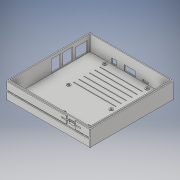
# Autodesk Inventor part: Tray
Saved by Autodesk Inventor 2018 (Build 220112000, 112)
## iProperties
Created: 2019-05-02
Part Number: Tray
Material: Generic
Document SubType Name: Modeling
Designer: thatg
Density: 1 g/cm^3
Appearance: Default
Author: thatg
Autodesk Inventor part; units mm, degrees
ref_plane "YZ Plane" through (0, 0, 0) normal (1, 0, 0) x (0, 1, 0)
ref_plane "XZ Plane" through (0, 0, 0) normal (0, 1, 0) x (-1, 0, 0)
ref_plane "XY Plane" through (0, 0, 0) normal (0, 0, 1) x (1, 0, 0)
sketch "Sketch1" plane through (0, 0, 0) normal (0, 1, 0) x (-1, 0, 0)
  line L0 (-57.15, 57.15) -> (57.15, 57.15)
  line L1 (57.15, 57.15) -> (57.15, -57.15)
  line L2 (57.15, -57.15) -> (-57.15, -57.15)
  line L3 (-57.15, -57.15) -> (-57.15, 57.15)
  line L4 (-57.15, 57.15) -> (57.15, -57.15) construction
  line L5 (57.15, 57.15) -> (-57.15, -57.15) construction
  point P0 (0, 0)
  dimension "d0" = 114.3
  dimension "d1" = 114.3
  constraints: 12 end point, 2 midpoint, 2 parallel, 1 horizontal, 1 perpendicular
  measures "d0" distance of L1.end L2.end
  measures "d1" distance of L0.end L1.end
extrude "Extrusion1" add sketch "Sketch1" along normal blind 2.54
sketch "Sketch4" plane through (0, 2.54, 0) normal (0, 1, 0) x (1, 0, 0)
  line L0 (-57.15, -57.15) -> (57.15, -57.15) projected
  line L1 (57.15, -57.15) -> (57.15, 57.15) projected
  line L2 (57.15, 57.15) -> (-57.15, 57.15) projected
  line L3 (-57.15, 57.15) -> (-57.15, -57.15) projected
  line L4 (-54.61, 54.61) -> (54.61, 54.61)
  line L5 (54.61, 54.61) -> (54.61, -54.61)
  line L6 (54.61, -54.61) -> (-54.61, -54.61)
  line L7 (-54.61, -54.61) -> (-54.61, 54.61)
  point P0 (0, 0)
  dimension "d11" = 2.54
  constraints: 8 end point, 3 other
  measures "d11" distance between parallel lines of L2 L4
extrude "Extrusion4" add sketch "Sketch4" along normal blind 20
sketch "Sketch6" plane through (0, 2.54, 0) normal (0, 1, 0) x (1, 0, 0)
  line L0 (-53.34, 53.34) -> (-53.34, -0.12)
  line L1 (-53.34, 53.34) -> (-53.34, -2.66)
  line L2 (-53.34, -2.66) -> (31.66, -2.66)
  line L3 (31.66, -2.66) -> (31.66, 53.34)
  line L4 (31.66, 53.34) -> (-53.34, 53.34)
  line L5 (-53.34, 53.34) -> (31.66, 53.34)
  line L6 (31.66, 53.34) -> (31.66, -2.66)
  line L7 (31.66, -2.66) -> (-53.34, -2.66)
  line L8 (-53.34, -2.66) -> (-53.34, 53.34)
  line L9 (-57.15, 8.34) -> (-54.61, 8.34)
  line L10 (-57.15, 24.34) -> (-54.61, 24.34)
  line L11 (-57.15, 43.09) -> (-54.61, 43.09)
  line L12 (-57.15, 53.34) -> (-53.34, 53.34)
  line L13 (-57.15, 14.915) -> (-54.61, 14.915)
  line L14 (-57.15, 1.765) -> (-54.61, 1.765)
  line L15 (-57.15, 30.915) -> (-54.61, 30.915)
  line L16 (-57.15, 17.765) -> (-54.61, 17.765)
  line L17 (-57.15, 51.065) -> (-54.61, 51.065)
  line L18 (-57.15, 35.115) -> (-54.61, 35.115)
  line L19 (-57.15, 51.065) -> (-54.61, 51.065)
  line L20 (-53.34, 51.065) -> (-53.34, 35.115)
  line L21 (-54.61, 35.115) -> (-57.15, 35.115)
  line L22 (-57.15, 35.115) -> (-57.15, 51.065)
  line L23 (-57.15, 30.915) -> (-54.61, 30.915)
  line L24 (-53.34, 30.915) -> (-53.34, 17.765)
  line L25 (-54.61, 17.765) -> (-57.15, 17.765)
  line L26 (-57.15, 17.765) -> (-57.15, 30.915)
  line L27 (-57.15, 14.915) -> (-54.61, 14.915)
  line L28 (-53.34, 14.915) -> (-53.34, 1.765)
  line L29 (-54.61, 1.765) -> (-57.15, 1.765)
  line L30 (-57.15, 1.765) -> (-57.15, 14.915)
  line L31 (31.66, 53.34) -> (31.66, 57.15)
  line L32 (21.06, 57.15) -> (21.06, 54.61)
  line L33 (17.06, 57.15) -> (17.06, 54.61)
  line L34 (25.06, 57.15) -> (25.06, 54.61)
  line L35 (-0.34, 57.15) -> (-0.34, 54.61)
  line L36 (7.41, 57.15) -> (7.41, 54.61)
  line L37 (-8.09, 57.15) -> (-8.09, 54.61)
  line L38 (-21.84, 57.15) -> (-21.84, 54.61)
  line L39 (-25.09, 57.15) -> (-25.09, 54.61)
  line L40 (-18.59, 57.15) -> (-18.59, 54.61)
  line L41 (-25.09, 57.15) -> (-18.59, 57.15)
  line L42 (-18.59, 57.15) -> (-18.59, 54.61)
  line L43 (-18.59, 53.34) -> (-25.09, 53.34)
  line L44 (-25.09, 54.61) -> (-25.09, 57.15)
  line L45 (-8.09, 57.15) -> (7.41, 57.15)
  line L46 (7.41, 57.15) -> (7.41, 54.61)
  line L47 (7.41, 53.34) -> (-8.09, 53.34)
  line L48 (-8.09, 54.61) -> (-8.09, 57.15)
  line L49 (17.06, 57.15) -> (25.06, 57.15)
  line L50 (25.06, 57.15) -> (25.06, 54.61)
  line L51 (25.06, 53.34) -> (17.06, 53.34)
  line L52 (17.06, 54.61) -> (17.06, 57.15)
  line L53 (-54.61, 54.61) -> (54.61, 54.61) projected
  line L54 (-25.09, 54.61) -> (-18.59, 54.61)
  line L55 (-8.09, 54.61) -> (7.41, 54.61)
  line L56 (17.06, 54.61) -> (25.06, 54.61)
  line L57 (-54.61, -54.61) -> (-54.61, 54.61) projected
  line L58 (-54.61, 51.065) -> (-54.61, 35.115)
  line L59 (-54.61, 30.915) -> (-54.61, 17.765)
  line L60 (-54.61, 14.915) -> (-54.61, 1.765)
  point P0 (0, 0)
  dimension "d17" = 56
  dimension "d18" = 85
  dimension "d21" = 10.25
  dimension "d22" = 18.75
  dimension "d23" = 16
  dimension "d24" = 6.575
  dimension "d25" = 6.575
  dimension "d26" = 6.575
  dimension "d27" = 6.575
  dimension "d28" = 7.975
  dimension "d29" = 7.975
  dimension "d30" = 10.6
  dimension "d31" = 4
  dimension "d32" = 4
  dimension "d33" = 21.4
  dimension "d34" = 7.75
  dimension "d35" = 7.75
  dimension "d37" = 21.5
  dimension "d38" = 3.25
  dimension "d39" = 3.25
  constraints: 118 end point, 26 parallel, 15 perpendicular, 9 horizontal, 6 point on line, 5 midpoint, 1 vertical, 8 other
  measures "d17" distance of L0.start L1.end
  measures "d18" distance of L1.end L2.end
  measures "d21" distance of L12.start L11.start
  measures "d22" distance of L11.start L10.start
  measures "d23" distance of L10.start L9.start
  measures "d24" distance between parallel lines of L9 L13
  measures "d25" distance between parallel lines of L9 L14
  measures "d26" distance between parallel lines of L10 L15
  measures "d27" distance between parallel lines of L10 L16
  measures "d28" distance between parallel lines of L11 L17
  measures "d29" distance between parallel lines of L11 L18
  measures "d30" distance of L31.end L32.start
  measures "d31" distance between parallel lines of L32 L33
  measures "d32" distance between parallel lines of L32 L34
  measures "d33" distance of L32.start L35.start
  measures "d34" distance between parallel lines of L35 L36
  measures "d35" distance between parallel lines of L35 L37
  measures "d37" distance of L35.start L38.start
  measures "d38" distance between parallel lines of L38 L39
  measures "d39" distance between parallel lines of L38 L40
extrude "Extrusion5" cut sketch "Sketch6" along normal blind 17.5 contours L30 L13 L57 L9 | L9 L57 L14 L30 | L26 L15 L57 L10 | L10 L57 L16 L26
extrude "Extrusion6" cut sketch "Sketch6" along normal blind 15 contours L22 L17 L57 L11 | L11 L57 L18 L22
extrude "Extrusion7" cut sketch "Sketch6" along normal blind 7.5 contours L39 L41 L38 L53 | L38 L41 L40 L53
extrude "Extrusion8" cut sketch "Sketch6" along normal blind 8 contours L37 L45 L35 L53 | L35 L45 L36 L53
extrude "Extrusion9" cut sketch "Sketch6" along normal blind 3.5 contours L53 L32 L49 L34 | L33 L49 L32 L53
sketch "Sketch7" plane through (0, 2.54, 0) normal (0, 1, 0) x (1, 0, 0)
  line L0 (-57.15, 1.765) -> (-57.15, 14.915) projected
  line L1 (-57.15, 1.765) -> (-54.61, 1.765) projected
  line L2 (-54.61, 14.915) -> (-57.15, 14.915) projected
  line L3 (-57.15, 17.765) -> (-54.61, 17.765) projected
  line L4 (-57.15, 17.765) -> (-57.15, 30.915) projected
  line L5 (-54.61, 30.915) -> (-57.15, 30.915) projected
  line L6 (-57.15, 35.115) -> (-54.61, 35.115) projected
  line L7 (-57.15, 35.115) -> (-57.15, 51.065) projected
  line L8 (-54.61, 51.065) -> (-57.15, 51.065) projected
  line L9 (-18.59, 54.61) -> (-18.59, 57.15) projected
  line L10 (-25.09, 57.15) -> (-18.59, 57.15) projected
  line L11 (-25.09, 57.15) -> (-25.09, 54.61) projected
  line L12 (-8.09, 57.15) -> (-8.09, 54.61) projected
  line L13 (-8.09, 57.15) -> (7.41, 57.15) projected
  line L14 (7.41, 54.61) -> (7.41, 57.15) projected
  line L15 (17.06, 57.15) -> (17.06, 54.61) projected
  line L16 (17.06, 57.15) -> (25.06, 57.15) projected
  line L17 (25.06, 54.61) -> (25.06, 57.15) projected
  line L18 (-54.61, 1.765) -> (-54.61, 14.915)
  line L19 (-54.61, 17.765) -> (-54.61, 30.915)
  line L20 (-54.61, 35.115) -> (-54.61, 51.065)
  line L21 (-25.09, 54.61) -> (-18.59, 54.61)
  line L22 (-8.09, 54.61) -> (7.41, 54.61)
  line L23 (17.06, 54.61) -> (25.06, 54.61)
  point P0 (0, 0)
  constraints: 12 end point, 4 collinear, 1 perpendicular, 1 vertical
extrude "Extrusion10" add sketch "Sketch7" along normal blind 1
sketch "Sketch8" plane through (0, 2.54, 0) normal (0, 1, 0) x (1, 0, 0)
  line L0 (-53.34, -2.66) -> (31.66, -2.66) projected
  line L1 (31.66, -2.66) -> (31.66, 53.34) projected
  line L2 (31.66, 53.34) -> (-53.34, 53.34) projected
  line L3 (-53.34, 53.34) -> (-53.34, -2.66) projected
  line L4 (31.66, -2.66) -> (28.16, -2.66)
  line L5 (28.16, -2.66) -> (28.16, 0.84)
  circle A0 centre (28.16, 0.84) radius 1.175
  line L6 (31.66, 53.34) -> (28.16, 53.34)
  line L7 (28.16, 53.34) -> (28.16, 49.84)
  circle A1 centre (28.16, 49.84) radius 1.175
  line L8 (28.16, 0.84) -> (-29.84, 0.84)
  circle A2 centre (-29.84, 0.84) radius 1.175
  line L9 (28.16, 49.84) -> (-29.84, 49.84)
  circle A3 centre (-29.84, 49.84) radius 1.175
  circle A4 centre (-29.84, 0.84) radius 2.445
  circle A5 centre (28.16, 0.84) radius 2.445
  circle A6 centre (28.16, 49.84) radius 2.445
  circle A7 centre (-29.84, 49.84) radius 2.445
  point P0 (0, 0)
  dimension "d52" = 3.5
  dimension "d53" = 3.5
  dimension "d54" = 2.35
  dimension "d56" = 3.5
  dimension "d57" = 3.5
  dimension "d58" = 2.35
  dimension "d59" = 58
  dimension "d60" = 2.35
  dimension "d61" = 58
  dimension "d62" = 2.35
  dimension "d63" = 1.27
  dimension "d64" = 1.27
  dimension "d65" = 1.27
  dimension "d66" = 1.27
  constraints: 12 end point, 8 centre point, 4 coincident, 2 perpendicular, 2 point on line, 1 horizontal, 1 parallel
  measures "d52" distance of L0.end L4.end
  measures "d53" distance of L4.end L5.end
  measures "d54" diameter of A0
  measures "d56" distance of L1.end L6.end
  measures "d57" distance of L6.end L7.end
  measures "d58" diameter of A1
  measures "d59" distance of L8.start L8.end
  measures "d60" diameter of A2
  measures "d61" distance of L9.start L9.end
  measures "d62" diameter of A3
  measures "d63" radial gap between concentric circles of A2 A4
  measures "d64" radial gap between concentric circles of A0 A5
  measures "d65" radial gap between concentric circles of A1 A6
  measures "d66" radial gap between concentric circles of A3 A7
extrude "Extrusion11" add sketch "Sketch8" along normal blind 0.5 contours A5 L8 A0 L5 | L5 A0 L8 A5 | A6 L9 A1 L7 | L7 A1 L9 A6 | A4 | A7
sketch "Sketch9" plane through (0, 2.54, 0) normal (0, 1, 0) x (1, 0, 0)
  circle A0 centre (28.16, 0.84) radius 1.175 projected
  circle A1 centre (-29.84, 0.84) radius 1.175 projected
  circle A2 centre (-29.84, 49.84) radius 1.175 projected
  circle A3 centre (28.16, 49.84) radius 1.175 projected
  point P0 (0, 0)
extrude "Extrusion12" cut sketch "Sketch9" against normal blind 1.905
thread "Thread1" size "M2.5x0.45" class "6H" standard "ANSI Metric M Profile" full length
thread "Thread2" size "M2.5x0.45" class "6H" standard "ANSI Metric M Profile" full length
thread "Thread3" size "M2.5x0.45" class "6H" standard "ANSI Metric M Profile" full length
thread "Thread4" size "M2.5x0.45" class "6H" standard "ANSI Metric M Profile" full length
sketch "Sketch10" plane through (57.15, 0, -57.15) normal (0, 0, -1) x (-1, 0, 0)
  line L0 (0, 22.54) -> (114.3, 22.54) projected
  line L1 (0, 0) -> (0, 22.54) projected
  line L2 (114.3, 0) -> (0, 0) projected
  line L3 (114.3, 0) -> (114.3, 22.54) projected
  line L4 (114.3, 20.635) -> (30.4644, 20.635)
  line L5 (30.4644, 1.905) -> (114.3, 1.905)
  line L6 (30.4644, 1.905) -> (30.4644, 20.635)
  line L7 (114.3, 20.635) -> (114.3, 1.905)
  line L8 (114.3, 0) -> (114.3, 22.54) projected
  point P0 (57.15, 0)
  point P1 (32.09, 3.54)
  point P2 (114.3, 20.04)
  dimension "d79" = 1.905
  dimension "d81" = 1.6256
  constraints: 8 end point, 2 point on line, 1 collinear, 1 perpendicular
  measures "d79" distance between parallel lines of L0 L4
  measures "d81" horizontal distance of L5.start point (32.09, 3.54)
extrude "Extrusion13" cut sketch "Sketch10" against normal blind 1.27 contours L3 L5 L6 L4
sketch "Sketch11" plane through (-57.15, 0, -57.15) normal (-1, 0, 0) x (0, 0, 1)
  line L0 (0, 22.54) -> (114.3, 22.54) projected
  line L1 (114.3, 0) -> (0, 0) projected
  line L2 (114.3, 0) -> (114.3, 22.54) projected
  line L3 (0, 20.635) -> (57.0106, 20.635)
  line L4 (112.395, 20.635) -> (112.395, 1.905)
  line L5 (57.0106, 1.905) -> (0, 1.905)
  line L6 (57.0106, 1.905) -> (57.0106, 20.635)
  line L7 (0, 20.635) -> (0, 1.905)
  line L8 (1.27, 20.635) -> (1.27, 1.905) projected
  point P0 (57.15, 0)
  point P1 (55.385, 3.54)
  dimension "d84" = 1.905
  dimension "d86" = 1.6256
  constraints: 10 end point, 1 parallel, 1 perpendicular
  measures "d84" distance between parallel lines of L0 L3
  measures "d86" distance from line of L6 point (55.385, 3.54)
extrude "Extrusion14" cut sketch "Sketch11" against normal blind 1.27
sketch "Sketch12" plane through (0, 22.54, 0) normal (0, 1, 0) x (1, 0, 0)
  line L0 (54.61, 54.61) -> (54.61, -54.61) projected
  line L1 (54.61, -54.61) -> (-54.61, -54.61) projected
  line L2 (-54.61, -54.61) -> (-54.61, 54.61) projected
  line L3 (-54.61, 54.61) -> (54.61, 54.61) projected
  line L4 (55.88, -55.88) -> (55.88, 55.88)
  line L5 (55.88, 55.88) -> (-55.88, 55.88)
  line L6 (-55.88, 55.88) -> (-55.88, -55.88)
  line L7 (-55.88, -55.88) -> (55.88, -55.88)
  point P0 (0, 0)
  dimension "d89" = 1.27
  constraints: 8 end point, 3 other
  measures "d89" distance between parallel lines of L0 L4
extrude "Extrusion15" add sketch "Sketch12" along normal blind 1.27
fillet "Fillet1" radius 1.27 20 edges at (-57.15, 0, 0) (0, 0, -57.15) (-57.15, 0.9525, -57.15) (-55.88, 11.27, -55.88) (-57.15, 21.5875, -57.15) (-55.88, 23.175, -55.88) (-54.61, 13.175, -54.61) (-57.15, 11.27, 57.15) (-55.88, 23.175, 55.88) (-54.61, 13.175, 54.61) (0, 0, 57.15) (57.15, 11.27, 57.15) (55.88, 23.175, 55.88) (54.61, 13.175, 54.61) (57.15, 0, 0) (57.15, 11.27, -57.15) (55.88, 23.175, -55.88) (54.61, 13.175, -54.61) (26.6856, 11.27, -57.15) (-57.15, 11.27, -0.1394)
sketch "Sketch13" plane through (-55.88, 1.27, 57.15) normal (0, 0, 1) x (1, 0, 0)
  line L0 (111.76, 0) -> (0, 0) projected
  line L1 (110.49, 11.43) -> (1.27, 11.43)
  line L2 (110.49, 9.525) -> (1.27, 9.525)
  line L3 (1.27, 11.43) -> (1.27, 9.525)
  line L4 (0, 2.27) -> (0, 16.27) projected
  line L5 (110.49, 11.43) -> (110.49, 9.525)
  line L6 (111.76, 0) -> (111.76, 21.27) projected
  point P0 (55.88, -1.27)
  dimension "d94" = 11.43
  dimension "d95" = 1.905
  dimension "d96" = 1.27
  dimension "d97" = 1.27
  constraints: 8 end point, 2 parallel, 2 vertical, 2 other
  measures "d94" distance between parallel lines of L0 L1
  measures "d95" distance between parallel lines of L1 L2
  measures "d96" distance of the line from the sketch origin of L3
extrude "Extrusion16" cut sketch "Sketch13" against normal blind 1.27
sketch "Sketch14" plane through (-55.88, 1.27, 55.88) normal (0, 0, 1) x (1, 0, 0)
  line L0 (1.27, 9.525) -> (1.27, 11.43) projected
  line L1 (5.715, 11.43) -> (5.715, 9.525)
  line L2 (1.27, 9.525) -> (1.27, 11.43)
  line L3 (5.715, 11.43) -> (10.16, 11.43)
  line L4 (10.16, 11.43) -> (10.16, 9.525)
  line L5 (10.16, 9.525) -> (5.715, 9.525)
  line L6 (5.715, 9.525) -> (5.715, 11.43)
  line L7 (110.49, 9.525) -> (1.27, 9.525) projected
  line L8 (55.88, 9.525) -> (55.88, 11.43)
  line L9 (1.27, 11.43) -> (110.49, 11.43) projected
  line L10 (110.49, 9.525) -> (110.49, 11.43)
  line L11 (106.045, 11.43) -> (106.045, 9.525)
  line L12 (110.49, 9.525) -> (110.49, 11.43)
  line L13 (106.045, 11.43) -> (101.6, 11.43)
  line L14 (101.6, 11.43) -> (101.6, 9.525)
  line L15 (101.6, 9.525) -> (106.045, 9.525)
  line L16 (106.045, 9.525) -> (106.045, 11.43)
  point P0 (55.88, -1.27)
  dimension "d100" = 4.445
  dimension "d101" = 4.445
  constraints: 28 end point, 7 symmetric about line, 3 parallel, 2 midpoint, 1 horizontal, 1 perpendicular
  measures "d100" distance of L1.end L2.start
  measures "d101" distance of L4.end L5.end
extrude "Extrusion17" cut sketch "Sketch14" against normal up to surface (1.27 mm away) contours L1 L3 L4 L5 | L14 L9 L11 L7
fillet "Fillet3" radius 1.27 2 edges at (-54.61, 11.7475, 57.15) (54.61, 11.7475, 57.15)
sketch "Sketch15" plane through (-55.88, 22.54, 57.15) normal (0, 0, 1) x (1, 0, 0)
  line L0 (101.6, -9.84) -> (99.3775, -9.84)
  line L1 (99.3775, -9.84) -> (99.3775, -4.76)
  line L2 (99.3775, -9.84) -> (104.4575, -9.84) construction
  line L3 (98.679, -4.76) -> (75.3775, -4.76)
  line L4 (75.3775, -4.0615) -> (98.679, -4.0615)
  line L5 (75.3775, -5.4585) -> (98.679, -5.4585)
  line L6 (75.3775, -4.0615) -> (75.3775, -5.4585)
  line L7 (98.679, -5.4585) -> (98.679, -4.0615)
  line L8 (111.76, 0) -> (111.76, -9.84) projected
  point P0 (55.88, -22.54)
  dimension "d105" = 2.2225
  dimension "d106" = 5.08
  dimension "d107" = 90
  dimension "d108" = 24
  dimension "d109" = 0.6985
  dimension "d110" = 0.6985
  dimension "d111" = 0.6985
  dimension "d112" = 23.3015
  constraints: 16 end point, 3 horizontal, 2 perpendicular, 2 vertical, 1 midpoint
  measures "d105" distance of L0.start L0.end
  measures "d106" distance of L0.end L1.end
  measures "d107" angle of L2 L1
  measures "d108" distance of L1.end L3.end
  measures "d109" distance between parallel lines of L3 L4
  measures "d110" distance between parallel lines of L3 L5
  measures "d111" distance of L1.end L3.start
  measures "d112" distance between parallel lines of L7 L6
extrude "Extrusion18" cut sketch "Sketch15" against normal up to surface (2.54 mm away)
sketch "Sketch16" plane through (-55.88, 22.54, 57.15) normal (0, 0, 1) x (1, 0, 0)
  line L0 (98.679, -4.0615) -> (75.3775, -4.0615) projected
  line L1 (87.0282, -9.84) -> (87.0282, 0)
  line L2 (110.49, 0) -> (1.27, 0) projected
  line L3 (0, -9.84) -> (111.76, -9.84) projected
  line L4 (80.6782, -9.84) -> (80.6782, -1.27)
  line L5 (93.3782, -9.84) -> (93.3782, -1.27)
  line L6 (80.6782, -9.84) -> (93.3782, -9.84)
  line L7 (101.6, -11.745) -> (10.16, -11.745) projected
  line L8 (81.9482, 0) -> (92.1082, 0)
  arc A0 (81.9482, 0) -> (80.6782, -1.27) centre (81.9482, -1.27) ccw
  arc A1 (93.3782, -1.27) -> (92.1082, 0) centre (92.1082, -1.27) ccw
  point P0 (55.88, -22.54)
  dimension "d117" = 6.35
  dimension "d118" = 6.35
  dimension "d119" = 1.27
  constraints: 10 end point, 4 point on circle, 4 tangent, 3 parallel, 2 centre point, 2 point on line, 1 collinear, 1 equal radius, 1 vertical
  measures "d117" distance between parallel lines of L1 L4
  measures "d118" distance between parallel lines of L1 L5
  measures "d119" radius of A0
extrude "Extrusion19" cut sketch "Sketch16" against normal blind 1.27
ref_plane "Work Plane1" through (31.1482, 12.7, 57.15) normal (1, 0, 0) x (0, 0, -1)
sketch "Sketch17" plane through (31.1482, 12.7, 57.15) normal (1, 0, 0) x (0, 0, -1)
  line L0 (1.27, 5.7785) -> (1.27, 8.57) projected
  line L1 (1.27, 5.7785) -> (1.27, 7.0485)
  line L2 (1.27, 5.7785) -> (1.905, 5.7785)
  line L3 (0, 5.7785) -> (2.54, 5.7785) projected
  line L4 (1.905, 5.7785) -> (1.27, 7.0485)
  line L5 (0, 4.3815) -> (2.54, 4.3815) projected
  line L6 (1.27, 4.3815) -> (1.905, 4.3815)
  line L7 (1.905, 4.3815) -> (1.905, 3.7465)
  line L8 (1.27, 4.3815) -> (1.27, 3.7465)
  line L9 (1.27, 0) -> (1.27, 4.3815) projected
  line L10 (1.27, 3.7465) -> (1.27, 1.8415)
  line L11 (1.27, 1.8415) -> (1.905, 3.7465)
  point P0 (57.15, -12.7)
  dimension "d122" = 1.27
  dimension "d123" = 0.635
  dimension "d124" = 0.635
  dimension "d125" = 0.635
  dimension "d126" = 0.635
  dimension "d127" = 1.905
  constraints: 16 end point, 5 point on line, 1 midpoint, 1 perpendicular
  measures "d122" distance of L0.start L1.end
  measures "d123" distance of L0.start L2.end
  measures "d124" distance of L6.start L6.end
  measures "d125" distance of L6.end L7.end
  measures "d126" distance of L6.start L8.end
  measures "d127" distance of L8.end L10.end
extrude "Extrusion20" cut sketch "Sketch17" along normal mid plane 7.62
sketch "Sketch18" plane through (27.3382, 17.0815, 55.245) normal (0, 0, 1) x (1, 0, 0)
  line L0 (0, 0) -> (7.62, 0) projected
  line L1 (0, 0) -> (0, -0.635) projected
  line L2 (0, -0.635) -> (7.62, -0.635) projected
  line L3 (7.62, -0.635) -> (7.62, 0) projected
  point P0 (-27.3382, -17.0815)
extrude "Extrusion21" cut sketch "Sketch18" against normal up to surface (0.635 mm away)
fillet "Fillet4" radius 1.27 2 edges at (19.4975, 17.78, 57.15) (42.799, 17.78, 57.15)
ref_plane "Work Plane2" through (0, 8.255, 0) normal (0, 1, 0) x (1, 0, 0)
sketch "Sketch19" plane through (0, 8.255, 0) normal (0, 1, 0) x (1, 0, 0)
  line L0 (50.165, -54.61) -> (45.72, -54.61) projected
  line L1 (50.165, -54.61) -> (52.705, -54.61)
  line L2 (-53.34, -54.61) -> (53.34, -54.61) projected
  line L3 (52.705, -54.61) -> (52.705, -52.07)
  line L4 (52.705, -52.07) -> (50.165, -52.07)
  line L5 (50.165, -52.07) -> (50.165, -52.705)
  line L6 (50.165, -52.705) -> (51.435, -52.705)
  line L7 (51.435, -52.705) -> (51.435, -54.61)
  line L8 (19.4975, -54.61) -> (27.3382, -54.61) projected
  line L9 (19.4975, -54.61) -> (16.9575, -54.61)
  line L10 (16.9575, -54.61) -> (16.9575, -52.07)
  line L11 (16.9575, -52.07) -> (19.4975, -52.07)
  line L12 (19.4975, -52.07) -> (19.4975, -52.705)
  line L13 (19.4975, -52.705) -> (18.2275, -52.705)
  line L14 (18.2275, -52.705) -> (18.2275, -54.61)
  point P0 (0, 0)
  dimension "d134" = 2.54
  dimension "d135" = 2.54
  dimension "d136" = 2.54
  dimension "d137" = 0.635
  dimension "d138" = 1.27
  dimension "d139" = 2.54
  dimension "d140" = 2.54
  dimension "d141" = 2.54
  dimension "d142" = 0.635
  dimension "d143" = 1.27
  constraints: 24 end point, 8 perpendicular, 2 midpoint, 2 point on line
  measures "d134" distance of L0.start L1.end
  measures "d135" distance of L1.end L3.end
  measures "d136" distance of L3.end L4.end
  measures "d137" distance of L4.end L5.end
  measures "d138" distance of L5.end L6.end
  measures "d139" distance of L8.start L9.end
  measures "d140" distance of L9.end L10.end
  measures "d141" distance of L10.end L11.end
  measures "d142" distance of L11.end L12.end
  measures "d143" distance of L12.end L13.end
extrude "Extrusion22" add sketch "Sketch19" along normal up to surface (14.285 mm away)
sketch "Sketch20" plane through (0, 8.255, 0) normal (0, -1, 0) x (1, 0, 0)
  line L0 (52.705, 52.07) -> (52.705, 54.61) projected
  line L1 (16.9575, 54.61) -> (16.9575, 52.07) projected
  line L2 (52.705, 54.61) -> (16.9575, 54.61)
  line L3 (53.34, 54.61) -> (-53.34, 54.61) projected
  line L4 (16.9575, 52.07) -> (52.705, 52.07)
  point P0 (0, 0)
  constraints: 4 end point, 1 collinear, 1 parallel
extrude "Extrusion23" add sketch "Sketch20" against normal blind 1.27
sketch "Sketch21" plane through (0, 9.525, 0) normal (0, 1, 0) x (1, 0, 0)
  line L0 (50.165, -52.705) -> (50.165, -52.07) projected
  line L1 (19.4975, -52.07) -> (19.4975, -52.705) projected
  line L2 (19.4975, -52.705) -> (50.165, -52.705)
  line L3 (50.165, -52.07) -> (19.4975, -52.07) projected
  line L4 (50.165, -52.07) -> (19.4975, -52.07)
  point P0 (0, 0)
  constraints: 4 end point, 2 horizontal
extrude "Extrusion24" add sketch "Sketch21" along normal blind 1.27
sketch "Sketch22" plane through (0, 9.525, 0) normal (0, 1, 0) x (1, 0, 0)
  line L0 (19.4975, -52.705) -> (50.165, -52.705) projected
  line L1 (34.8313, -52.705) -> (34.8313, -54.61)
  line L2 (53.34, -54.61) -> (-53.34, -54.61) projected
  line L3 (36.1013, -52.705) -> (36.1013, -54.61)
  line L4 (33.5613, -52.705) -> (33.5613, -54.61)
  line L5 (36.1013, -54.61) -> (33.5613, -54.61)
  line L6 (33.5613, -52.705) -> (36.1013, -52.705)
  point P0 (0, 0)
  dimension "d150" = 1.27
  dimension "d151" = 1.27
  constraints: 10 end point, 2 parallel, 1 collinear, 1 horizontal, 1 midpoint, 1 point on line, 1 vertical
  measures "d150" distance between parallel lines of L1 L3
  measures "d151" distance between parallel lines of L1 L4
extrude "Extrusion25" cut sketch "Sketch22" against normal up to surface (1.27 mm away)
sketch "Sketch23" plane through (0, 2.54, 0) normal (0, 1, 0) x (1, 0, 0)
  circle A0 centre (28.16, 0.84) radius 2.445 projected
  circle A1 centre (-29.84, 49.84) radius 1.175 projected
  line L0 (28.16, 0.84) -> (-29.84, 0.84)
  line L1 (-29.84, 49.84) -> (28.16, 49.84)
  line L2 (27.8425, 7.19) -> (-29.5225, 7.19)
  line L3 (-29.5225, 43.49) -> (27.8425, 43.49)
  line L4 (27.8425, 7.825) -> (-29.5225, 7.825)
  line L5 (-29.5225, 42.855) -> (27.8425, 42.855)
  line L6 (27.8425, 14.175) -> (-29.5225, 14.175)
  line L7 (27.8425, 14.81) -> (-29.5225, 14.81)
  line L8 (-29.5225, 36.505) -> (27.8425, 36.505)
  line L9 (-29.5225, 35.87) -> (27.8425, 35.87)
  line L10 (27.8425, 21.16) -> (-29.5225, 21.16)
  line L11 (27.8425, 21.795) -> (-29.5225, 21.795)
  line L12 (-29.5225, 29.52) -> (27.8425, 29.52)
  line L13 (-29.5225, 28.885) -> (27.8425, 28.885)
  line L14 (28.16, 7.5075) -> (28.16, 7.5075)
  line L15 (28.16, 14.4925) -> (28.16, 14.4925)
  line L16 (28.16, 21.4775) -> (28.16, 21.4775)
  line L17 (28.16, 29.2025) -> (28.16, 29.2025)
  line L18 (28.16, 36.1875) -> (28.16, 36.1875)
  line L19 (28.16, 43.1725) -> (28.16, 43.1725)
  line L20 (-29.84, 7.5075) -> (-29.84, 7.5075)
  line L21 (-29.84, 14.4925) -> (-29.84, 14.4925)
  line L22 (-29.84, 21.4775) -> (-29.84, 21.4775)
  line L23 (-29.84, 29.2025) -> (-29.84, 29.2025)
  line L24 (-29.84, 36.1875) -> (-29.84, 36.1875)
  line L25 (-29.84, 43.1725) -> (-29.84, 43.1725)
  arc A2 (28.16, 7.5075) -> (27.8425, 7.825) centre (27.8425, 7.5075) ccw
  arc A3 (27.8425, 7.19) -> (28.16, 7.5075) centre (27.8425, 7.5075) ccw
  arc A4 (-29.84, 7.5075) -> (-29.5225, 7.19) centre (-29.5225, 7.5075) ccw
  arc A5 (-29.5225, 7.825) -> (-29.84, 7.5075) centre (-29.5225, 7.5075) ccw
  arc A6 (-29.84, 14.4925) -> (-29.5225, 14.175) centre (-29.5225, 14.4925) ccw
  arc A7 (-29.5225, 14.81) -> (-29.84, 14.4925) centre (-29.5225, 14.4925) ccw
  arc A8 (-29.84, 21.4775) -> (-29.5225, 21.16) centre (-29.5225, 21.4775) ccw
  arc A9 (-29.5225, 21.795) -> (-29.84, 21.4775) centre (-29.5225, 21.4775) ccw
  arc A10 (-29.84, 29.2025) -> (-29.5225, 28.885) centre (-29.5225, 29.2025) ccw
  arc A11 (-29.5225, 29.52) -> (-29.84, 29.2025) centre (-29.5225, 29.2025) ccw
  arc A12 (-29.84, 36.1875) -> (-29.5225, 35.87) centre (-29.5225, 36.1875) ccw
  arc A13 (-29.5225, 36.505) -> (-29.84, 36.1875) centre (-29.5225, 36.1875) ccw
  arc A14 (-29.84, 43.1725) -> (-29.5225, 42.855) centre (-29.5225, 43.1725) ccw
  arc A15 (-29.5225, 43.49) -> (-29.84, 43.1725) centre (-29.5225, 43.1725) ccw
  arc A16 (27.8425, 42.855) -> (28.16, 43.1725) centre (27.8425, 43.1725) ccw
  arc A17 (28.16, 43.1725) -> (27.8425, 43.49) centre (27.8425, 43.1725) ccw
  arc A18 (28.16, 36.1875) -> (27.8425, 36.505) centre (27.8425, 36.1875) ccw
  arc A19 (27.8425, 35.87) -> (28.16, 36.1875) centre (27.8425, 36.1875) ccw
  arc A20 (28.16, 29.2025) -> (27.8425, 29.52) centre (27.8425, 29.2025) ccw
  arc A21 (27.8425, 28.885) -> (28.16, 29.2025) centre (27.8425, 29.2025) ccw
  arc A22 (28.16, 21.4775) -> (27.8425, 21.795) centre (27.8425, 21.4775) ccw
  arc A23 (27.8425, 21.16) -> (28.16, 21.4775) centre (27.8425, 21.4775) ccw
  arc A24 (28.16, 14.4925) -> (27.8425, 14.81) centre (27.8425, 14.4925) ccw
  arc A25 (27.8425, 14.175) -> (28.16, 14.4925) centre (27.8425, 14.4925) ccw
  point P0 (0, 0)
  dimension "d154" = 6.35
  dimension "d155" = 6.35
  dimension "d156" = 0.635
  dimension "d157" = 0.635
  dimension "d158" = 6.35
  dimension "d159" = 0.635
  dimension "d160" = 6.35
  dimension "d161" = 0.635
  dimension "d162" = 6.35
  dimension "d163" = 0.635
  dimension "d164" = 6.35
  dimension "d165" = 0.635
  dimension "d166" = 0.3175
  dimension "d167" = 0.3175
  constraints: 52 end point, 48 point on circle, 48 tangent, 24 centre point, 22 equal radius, 14 parallel, 10 collinear, 1 horizontal, 1 vertical
  measures "d154" distance between parallel lines of L0 L2
  measures "d155" distance between parallel lines of L1 L3
  measures "d156" distance between parallel lines of L2 L4
  measures "d157" distance between parallel lines of L3 L5
  measures "d158" distance between parallel lines of L4 L6
  measures "d159" distance between parallel lines of L6 L7
  measures "d160" distance between parallel lines of L5 L8
  measures "d161" distance between parallel lines of L8 L9
  measures "d162" distance between parallel lines of L7 L10
  measures "d163" distance between parallel lines of L10 L11
  measures "d164" distance between parallel lines of L9 L12
  measures "d165" distance between parallel lines of L12 L13
  measures "d166" radius of A2
  measures "d167" radius of A5
extrude "Extrusion26" cut sketch "Sketch23" against normal up to surface (2.54 mm away) contours L2 A4 A5 L4 A2 A3 | L3 A17 A16 L5 A14 A15 | L6 A6 A7 L7 A24 A25 | L8 A18 A19 L9 A12 A13 | L10 A8 A9 L11 A22 A23 | L12 A20 A21 L13 A10 A11
body "Solid1"
